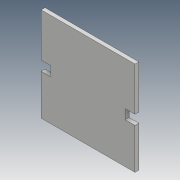
# Autodesk Inventor part: tapa
Saved by Autodesk Inventor 2017 (Build 210142000, 142)
## iProperties
Created: 2020-06-11
Part Number: tapa
Material: Generic
Document SubType Name: Modeling
Designer: c
Density: 1 g/cm^3
Appearance: Default
Author: c
Autodesk Inventor part; units mm, degrees
ref_plane "YZ Plane" through (0, 0, 0) normal (1, 0, 0) x (0, 1, 0)
ref_plane "XZ Plane" through (0, 0, 0) normal (0, 1, 0) x (-1, 0, 0)
ref_plane "XY Plane" through (0, 0, 0) normal (0, 0, 1) x (1, 0, 0)
sketch "Sketch1" plane through (0, 0, 0) normal (0, 1, 0) x (-1, 0, 0)
  line L0 (12, 19) -> (-37, 19)
  line L1 (-37, 19) -> (-37, -30)
  line L2 (-37, -30) -> (12, -30)
  line L3 (12, -30) -> (12, 19)
  point P0 (0, 0)
  dimension "d0" = 49
  dimension "d1" = 49
  constraints: 8 end point, 2 parallel, 1 horizontal, 1 perpendicular
  measures "d0" distance of L2.end L1.end
  measures "d1" distance of L1.end L0.end
extrude "Extrusion1" add sketch "Sketch1" along normal blind 2
sketch "Sketch5" plane through (0, 0, 0) normal (0, -1, 0) x (1, 0, 0)
  line L0 (43.3226, -3.7217) -> (43.3226, -8.7217)
  line L1 (-14.8869, -8.7217) -> (-14.8869, -3.7217)
  line L2 (-7, 21.3686) -> (32, 21.3686)
  line L3 (32, 21.3686) -> (32, -31.9902)
  line L4 (32, -31.9902) -> (-7, -31.9902)
  line L5 (-7, -31.9902) -> (-7, -3.7217)
  line L6 (37, 19) -> (37, -30) projected
  line L7 (-14.8869, -3.7217) -> (-7, -3.7217)
  line L8 (32, -3.7217) -> (43.3226, -3.7217)
  line L9 (43.3226, -8.7217) -> (32, -8.7217)
  line L10 (-7, -8.7217) -> (-14.8869, -8.7217)
  point P0 (0, 0)
  dimension "d39" = 5
  dimension "d40" = 39
  dimension "d41" = 5
  constraints: 20 end point, 7 parallel, 3 horizontal, 3 perpendicular, 3 point on line
  measures "d39" distance of L0.start L0.end
  measures "d40" distance of L2.start L2.end
  measures "d41" distance between parallel lines of L6 L3
extrude "Extrusion4" cut sketch "Sketch5" against normal blind 10
body "Solid1"
